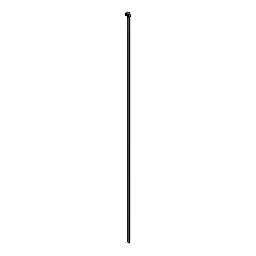
36part (Autodesk Fusion 360 design; units mm, degrees)
Autodesk Fusion 360 part; units mm, degrees
sketch "Sketch1" plane through (0, 0, 0) normal (1, 0, 0) x (0, 0, -1)
  line L0 (0, -270) -> (0, 0)
  dimension "d15" = 270
  constraint vertical L0
  constraint coincident L0.end origin
  measures "d15" distance of L0.start L0.end
sketch "Sketch2" plane through (0, 0, 0) normal (0, 1, 0) x (1, 0, 0)
  line L0 (-6, 3) -> (-3, 3)
  line L1 (-3, 3) -> (-3, 2)
  line L2 (-3, 2) -> (-6, 2)
  line L3 (-6, 2) -> (-6, 3)
  dimension "d1" = 1
  dimension "d2" = 3
  constraint horizontal L0
  constraint vertical L1
  constraint horizontal L2
  constraint vertical L3
  measures "d1" distance of L0.end L1.end
  measures "d2" distance of L0.start L0.end
sweep "Sweep1" add profiles "Sketch2" path "Sketch1" along L0 section 1
sketch "Sketch3" plane through (0, 0, 0) normal (0, 0, 1) x (1, 0, 0)
  line L0 (-6.7324, 2.9105) -> (-2.2324, 2.9105)
  line L1 (-2.2324, 2.9105) -> (-2.2324, -0.0895)
  line L2 (-2.2324, -0.0895) -> (-6.7324, -0.0895)
  line L3 (-6.7324, -0.0895) -> (-6.7324, 2.9105)
  line L4 (-5.9523, 1.9141) -> (-2.9523, 1.9141)
  line L5 (-2.9523, 1.9141) -> (-2.9523, 0.9141)
  line L6 (-2.9523, 0.9141) -> (-5.9523, 0.9141)
  line L7 (-5.9523, 0.9141) -> (-5.9523, 1.9141)
  dimension "d9" = 3
  dimension "d10" = 1
  dimension "d11" = 3
  dimension "d12" = 4.5
  constraint horizontal L0
  constraint vertical L1
  constraint horizontal L2
  constraint vertical L3
  constraint horizontal L4
  constraint vertical L5
  constraint horizontal L6
  constraint vertical L7
  measures "d9" distance of L4.start L4.end
  measures "d10" distance of L4.start L6.end
  measures "d11" distance of L0.start L2.end
  measures "d12" distance of L0.start L0.end
extrude "Extrude1" add sketch "Sketch3" against normal blind 3
